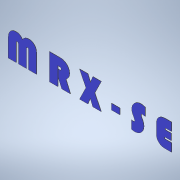
# Autodesk Inventor part: Logo
Saved by Autodesk Inventor 2021.2 (Build 252289000, 289)
## iProperties
Created: 2026-06-08
Part Number: Logo
Material: Generic
Document SubType Name: Modeling
Designer: NELSON
Density: 1 g/cm^3
Appearance: Default
Author: NELSON
Autodesk Inventor part; units mm, degrees
ref_plane "YZ Plane" through (0, 0, 0) normal (1, 0, 0) x (0, 1, 0)
ref_plane "XZ Plane" through (0, 0, 0) normal (0, 1, 0) x (-1, 0, 0)
ref_plane "XY Plane" through (0, 0, 0) normal (0, 0, 1) x (1, 0, 0)
sketch "Boceto1" plane through (0, 0, 0) normal (0, 0, 1) x (1, 0, 0)
  line L0 (-10.159, 4.8662) -> (417.1829, 4.8662) construction
  line L1 (417.1829, 4.8662) -> (417.1829, -72.825) construction
  line L2 (417.1829, -72.825) -> (-10.159, -72.825) construction
  line L3 (-10.159, -72.825) -> (-10.159, 4.8662) construction
  line L4 (38.6726, -55.1338) -> (38.6726, -17.2772)
  spline S0 degree 2 poles (38.6726, -17.2772) (38.6726, -14.5214) (37.5606, -12.8775) (36.2069, -12.8775) knots 0 0 0 1 2 2 2
  spline S1 degree 2 poles (36.2069, -12.8775) (34.7081, -12.8775) (33.4994, -14.5697) (33.4994, -17.2772) knots 0 0 0 1 2 2 2
  line L5 (33.4994, -17.2772) -> (33.4994, -55.1338)
  line L6 (33.4994, -55.1338) -> (15.6106, -55.1338)
  line L7 (15.6106, -55.1338) -> (15.6106, -17.2772)
  spline S2 degree 2 poles (15.6106, -17.2772) (15.6106, -14.5214) (14.4986, -12.8775) (13.1448, -12.8775) knots 0 0 0 1 2 2 2
  spline S3 degree 2 poles (13.1448, -12.8775) (11.646, -12.8775) (10.4373, -14.5697) (10.4373, -17.2772) knots 0 0 0 1 2 2 2
  line L8 (10.4373, -17.2772) -> (10.4373, -55.1338)
  line L9 (10.4373, -55.1338) -> (-7.2581, -55.1338)
  line L10 (-7.2581, -55.1338) -> (-7.2581, -17.664)
  spline S4 degree 2 poles (-7.2581, -17.664) (-7.2581, -11.7655) (-6.0494, -5.577) (-4.5989, -3.1596) knots 0 0 0 1 2 2 2
  spline S5 degree 2 poles (-4.5989, -3.1596) (-2.2782, 0.7083) (5.4091, 4.8662) (10.1956, 4.8662) knots 0 0 0 1 2 2 2
  spline S6 degree 2 poles (10.1956, 4.8662) (14.982, 4.8662) (22.7661, 0.3215) (24.555, -3.4496) knots 0 0 0 1 2 2 2
  spline S7 degree 2 poles (24.555, -3.4496) (26.3922, 0.3699) (34.0795, 4.8662) (38.866, 4.8662) knots 0 0 0 1 2 2 2
  spline S8 degree 2 poles (38.866, 4.8662) (43.0723, 4.8662) (50.0828, 1.7236) (52.4518, -1.3223) knots 0 0 0 1 2 2 2
  spline S9 degree 2 poles (52.4518, -1.3223) (54.5791, -3.9331) (56.4164, -10.8953) (56.4164, -17.664) knots 0 0 0 1 2 2 2
  line L11 (56.4164, -17.664) -> (56.4164, -55.1338)
  line L12 (56.4164, -55.1338) -> (38.6726, -55.1338)
  line L13 (105.3446, -20.4682) -> (108.0038, -20.4682)
  spline S10 degree 2 poles (108.0038, -20.4682) (110.2278, -20.4682) (111.8716, -19.0177) (111.8716, -17.2289) knots 0 0 0 1 2 2 2
  spline S11 degree 2 poles (111.8716, -17.2289) (111.8716, -15.5367) (110.4212, -14.2796) (108.0038, -14.2796) knots 0 0 0 1 2 2 2
  line L14 (108.0038, -14.2796) -> (104.3293, -14.2796)
  line L15 (104.3293, -14.2796) -> (104.3293, -55.1338)
  line L16 (104.3293, -55.1338) -> (85.5703, -55.1338)
  line L17 (85.5703, -55.1338) -> (85.5703, 3.7059)
  line L18 (85.5703, 3.7059) -> (107.3753, 3.7059)
  spline S12 degree 2 poles (107.3753, 3.7059) (113.3704, 3.7059) (119.7524, 1.7719) (122.7016, -0.3554) knots 0 0 0 1 2 2 2
  spline S13 degree 2 poles (122.7016, -0.3554) (126.6178, -3.2563) (130.8724, -11.6688) (130.8724, -16.4069) knots 0 0 0 1 2 2 2
  spline S14 degree 2 poles (130.8724, -16.4069) (130.8724, -21) (126.7629, -28.5907) (122.8467, -31.4915) knots 0 0 0 1 2 2 2
  line L19 (122.8467, -31.4915) -> (132.8064, -55.1338)
  line L20 (132.8064, -55.1338) -> (113.4188, -55.1338)
  line L21 (113.4188, -55.1338) -> (105.3446, -36.5198)
  line L22 (105.3446, -36.5198) -> (105.3446, -20.4682)
  line L23 (153.451, 3.7059) -> (172.2101, 3.7059)
  line L24 (172.2101, 3.7059) -> (177.8668, -9.9766)
  line L25 (177.8668, -9.9766) -> (183.3785, 3.7059)
  line L26 (183.3785, 3.7059) -> (202.2826, 3.7059)
  line L27 (202.2826, 3.7059) -> (187.7298, -25.7381)
  line L28 (187.7298, -25.7381) -> (202.2826, -55.1338)
  line L29 (202.2826, -55.1338) -> (183.4268, -55.1338)
  line L30 (183.4268, -55.1338) -> (177.8668, -41.4029)
  line L31 (177.8668, -41.4029) -> (172.2101, -55.1338)
  line L32 (172.2101, -55.1338) -> (153.451, -55.1338)
  line L33 (153.451, -55.1338) -> (167.9071, -25.7381)
  line L34 (167.9071, -25.7381) -> (153.451, 3.7059)
  line L35 (225.6347, -40.2909) -> (225.6347, -27.1402)
  line L36 (225.6347, -27.1402) -> (244.3938, -27.1402)
  line L37 (244.3938, -27.1402) -> (244.3938, -40.2909)
  line L38 (244.3938, -40.2909) -> (225.6347, -40.2909)
  line L39 (270.3567, -55.0854) -> (270.3567, -37.39)
  spline S15 degree 2 poles (270.3567, -37.39) (272.5324, -37.6801) (273.7895, -37.8252) (274.3213, -37.8252) knots 0 0 0 1 2 2 2
  spline S16 degree 2 poles (274.3213, -37.8252) (276.0618, -37.8252) (277.9957, -35.9879) (277.9957, -34.3441) knots 0 0 0 1 2 2 2
  spline S17 degree 2 poles (277.9957, -34.3441) (277.9957, -32.3618) (276.0618, -29.2675) knots 0 0 0 1 1 1
  spline S18 degree 2 poles (276.0618, -29.2675) (275.8201, -28.8808) (275.7717, -28.7357) knots 0 0 0 1 1 1
  spline S19 degree 2 poles (275.7717, -28.7357) (275.5783, -28.4456) (275.8201, -28.494) knots 0 0 0 1 1 1
  spline S20 degree 2 poles (275.8201, -28.494) (271.227, -21.4351) (271.227, -15.6817) knots 0 0 0 1 1 1
  spline S21 degree 2 poles (271.227, -15.6817) (271.227, -7.4625) (283.3624, 4.8662) (291.8233, 4.8662) knots 0 0 0 1 2 2 2
  spline S22 degree 2 poles (291.8233, 4.8662) (293.8539, 4.8662) (298.3503, 3.9476) (301.3962, 2.8356) knots 0 0 0 1 2 2 2
  line L40 (301.3962, 2.8356) -> (301.3962, -15.0532)
  spline S23 degree 2 poles (301.3962, -15.0532) (298.7854, -14.3763) (296.6581, -13.8445) (295.7878, -13.8445) knots 0 0 0 1 2 2 2
  spline S24 degree 2 poles (295.7878, -13.8445) (294.2407, -13.8445) (292.2584, -15.7784) (292.2584, -17.3739) knots 0 0 0 1 2 2 2
  spline S25 degree 2 poles (292.2584, -17.3739) (292.2584, -18.9694) (294.144, -22.112) knots 0 0 0 1 1 1
  spline S26 degree 2 poles (294.144, -22.112) (294.5308, -22.8372) (294.6275, -22.9823) knots 0 0 0 1 1 1
  spline S27 degree 2 poles (294.6275, -22.9823) (296.6098, -26.3183) (298.3986, -32.5552) (298.3986, -35.6978) knots 0 0 0 1 2 2 2
  spline S28 degree 2 poles (298.3986, -35.6978) (298.3986, -44.5455) (286.4567, -56.3425) (277.754, -56.3425) knots 0 0 0 1 2 2 2
  spline S29 degree 2 poles (277.754, -56.3425) (276.1585, -56.3425) (273.0642, -55.859) (270.3567, -55.0854) knots 0 0 0 1 2 2 2
  line L41 (360.816, -55.1338) -> (348.1005, -55.1338)
  spline S30 degree 2 poles (348.1005, -55.1338) (343.5558, -55.1338) (338.2375, -53.9734) (335.8684, -52.7164) knots 0 0 0 1 2 2 2
  spline S31 degree 2 poles (335.8684, -52.7164) (331.7105, -50.444) (327.0691, -43.0951) (327.0691, -38.8888) knots 0 0 0 1 2 2 2
  line L42 (327.0691, -38.8888) -> (327.0691, -17.4706)
  spline S32 degree 2 poles (327.0691, -17.4706) (327.0691, -10.1217) (329.8733, -3.2563) (333.3543, -0.4521) knots 0 0 0 1 2 2 2
  spline S33 degree 2 poles (333.3543, -0.4521) (335.9651, 1.7236) (343.4107, 3.7059) (349.0191, 3.7059) knots 0 0 0 1 2 2 2
  line L43 (349.0191, 3.7059) -> (360.816, 3.7059)
  line L44 (360.816, 3.7059) -> (360.816, -14.6181)
  line L45 (360.816, -14.6181) -> (349.1158, -14.6181)
  spline S34 degree 2 poles (349.1158, -14.6181) (347.472, -14.6181) (346.5534, -15.3916) (346.5534, -16.4069) knots 0 0 0 1 2 2 2
  spline S35 degree 2 poles (346.5534, -16.4069) (346.5534, -17.6156) (347.617, -18.5343) (349.1158, -18.5343) knots 0 0 0 1 2 2 2
  line L46 (349.1158, -18.5343) -> (360.0908, -18.5343)
  line L47 (360.0908, -18.5343) -> (360.0908, -32.8936)
  line L48 (360.0908, -32.8936) -> (347.472, -32.8936)
  spline S36 degree 2 poles (347.472, -32.8936) (345.9248, -32.8936) (345.0062, -33.6672) (345.0062, -34.6825) knots 0 0 0 1 2 2 2
  spline S37 degree 2 poles (345.0062, -34.6825) (345.0062, -35.9396) (346.0215, -36.8098) (347.472, -36.8098) knots 0 0 0 1 2 2 2
  line L49 (347.472, -36.8098) -> (360.816, -36.8098)
  line L50 (360.816, -36.8098) -> (360.816, -55.1338)
  point P0 (0, 0)
  constraints: 2 other
extrude "Extrusión1" add sketch "Boceto1" along normal blind 0.6
